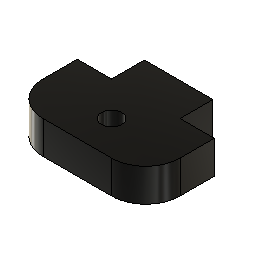
ThrowerLock v1 (Autodesk Fusion 360 design; units mm, degrees)
Autodesk Fusion 360 part; units mm, degrees
sketch "Sketch1" plane through (0, 0, 0) normal (0, 0, 1) x (1, 0, 0)
  line L0 (-5, 9.8) -> (5, 9.8)
  line L1 (5, 9.8) -> (5, 5)
  line L2 (5, 5) -> (10, 5)
  line L3 (10, 5) -> (10, 0)
  line L4 (5, -5) -> (-5, -5)
  line L5 (-10, 0) -> (-10, 5)
  line L6 (-10, 5) -> (-5, 5)
  line L7 (-5, 5) -> (-5, 9.8)
  line L8 (0, 0) -> (0, 9.8) construction
  line L9 (0, 0) -> (10, 0) construction
  line L10 (0, 0) -> (0, -5) construction
  line L11 (-5, 5) -> (-5, 0) construction
  line L12 (0, 0) -> (-5, 0) construction
  circle A0 centre (0, 0) radius 1.5
  line L13 (-10, -5) -> (-10, 0) construction
  line L14 (-5, -5) -> (-10, -5) construction
  arc A1 (-5, -5) -> (-10, 0) centre (-5, 0) ccw construction
  arc A2 (-10, 0) -> (-5, -5) centre (-5, 0) ccw
  line L15 (10, -5) -> (5, -5) construction
  line L16 (10, 0) -> (10, -5) construction
  arc A3 (10, 0) -> (5, -5) centre (5, 0) ccw construction
  arc A4 (5, -5) -> (10, 0) centre (5, 0) ccw
  point P0 (0, 9.8)
  point P1 (0, -5)
  point P2 (5, 0)
  dimension "d1" = 10
  dimension "d2" = 5
  dimension "d3" = 4.8
  dimension "d5" = 3
  dimension "d6" = 10
  constraint horizontal L0
  constraint perpendicular L0 L1
  constraint perpendicular L1 L2
  constraint perpendicular L2 L3
  constraint perpendicular L1 L4
  constraint perpendicular L4 L5
  constraint perpendicular L5 L6
  constraint vertical L7
  constraint collinear L2 L6
  constraint midpoint L0 P0
  constraint coincident L8.start L9.start
  constraint coincident L0 P0
  constraint perpendicular L0 L8
  constraint coincident L3 L9.end
  constraint perpendicular L3 L9
  constraint coincident P0 L8.end
  constraint coincident L3.end L9.end
  constraint coincident L4 P1
  constraint perpendicular L4 L10
  constraint coincident P1 L10.end
  constraint perpendicular L6 L11
  constraint perpendicular L11 L12
  constraint coincident L11.end L12.end
  constraint tangent L4 A1
  constraint midpoint L9 P2
  constraint coincident P2 A3.centre
  constraint tangent L4 A3
  constraint perpendicular L4 L13
  constraint perpendicular L1 L14
  constraint tangent L14 A3
  constraint concentric A1 A2
  constraint perpendicular L1 L15
  constraint concentric A3 A4
  constraint parallel L3 L16
  constraint tangent L13 A2
  measures "d1" distance of L0.start L0.end
  measures "d2" distance of L1.end L2.end
  measures "d3" distance of L0.start L6.end
  measures "d5" diameter of A0
  measures "d6" distance of L4 L6
extrude "Extrude1" add sketch "Sketch1" along normal blind 4.8
